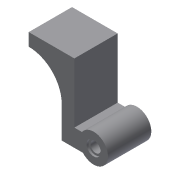
# Autodesk Inventor part: goal holder 2 flipped
Saved by Autodesk Inventor 2015 (Build 190159000, 159)
## iProperties
Created: 2014-11-06
Part Number: goal holder 2 flipped
Material: Generic
Document SubType Name: Modeling
Designer: jesse
Density: 1 g/cm^3
Appearance: Default
Author: jesse
Autodesk Inventor part; units mm, degrees
ref_plane "YZ Plane" through (0, 0, 0) normal (1, 0, 0) x (0, 1, 0)
ref_plane "XZ Plane" through (0, 0, 0) normal (0, 1, 0) x (-1, 0, 0)
ref_plane "XY Plane" through (0, 0, 0) normal (0, 0, 1) x (1, 0, 0)
sketch "Sketch1" plane through (0, 0, 0) normal (0, 0, 1) x (1, 0, 0)
  circle A0 centre (0, 0) radius 11 projected
  circle A1 centre (0, 0) radius 1.75 projected
  circle A2 centre (-8, 0) radius 1.75 projected
  circle A3 centre (0, 8) radius 1.75 projected
  circle A4 centre (8, 0) radius 1.75 projected
  circle A5 centre (0, -8) radius 1.75 projected
extrude "Extrusion1" add sketch "Sketch1" along normal blind 9.525
sketch "Sketch2" plane through (0, 0, 9.525) normal (0, 0, 1) x (1, 0, 0)
  circle A0 centre (0, 0) radius 11 projected
  line L0 (9.0377, 6.2705) -> (14.8574, 6.2705)
  line L1 (14.8574, 6.2705) -> (14.8574, 19.7717)
  line L2 (22.8575, 52.3603) -> (24.5877, 52.3603)
  line L3 (24.5877, 52.3603) -> (24.5877, -7.2164)
  line L4 (24.5877, -7.2164) -> (8.302, -7.2164)
  line L5 (22.8575, 52.3603) -> (14.8574, 52.3603)
  line L6 (14.8574, 19.7717) -> (14.8574, 52.3603)
  point P0 (-11, -11)
  dimension "d11" = 59.5767
  constraints: 14 end point, 3 horizontal, 3 perpendicular, 2 point on circle, 1 parallel, 1 vertical
  measures "d11" distance of L2.end L3.end
extrude "Extrusion2" add sketch "Sketch2" along normal blind 23.8125
mirror "Mirror1" about plane through (0, 0, 0) normal (1, 0, 0) remove original yes
sketch "Sketch3" plane through (-24.5877, -7.2164, 33.3375) normal (0, 0, 1) x (1, 0, 0)
  circle A0 centre (24.5877, 7.2164) radius 3.9688
  dimension "d4" = 7.9375
  constraints: 1 centre point, 1 coincident
  measures "d4" diameter of A0
extrude "Extrusion3" cut sketch "Sketch3" against normal blind 12.4
sketch "Sketch4" plane through (-24.5877, -7.2164, 33.3375) normal (0, 0, 1) x (1, 0, 0)
  circle A0 centre (24.5877, 7.2164) radius 5.5
  dimension "d7" = 11
  constraints: 1 centre point, 1 coincident
  measures "d7" diameter of A0
extrude "Extrusion4" cut sketch "Sketch4" against normal blind 1.5
mirror "Mirror2" about plane through (0, 0, 0) normal (1, 0, 0) remove original yes
sketch "Sketch7" plane through (24.5877, -7.2164, 9.525) normal (1, 0, 0) x (0, 0, -1)
  line L0 (0, 0) -> (0, 59.5767) projected
  line L1 (0, 59.5767) -> (-23.8125, 59.5767) projected
  line L2 (-23.8125, 0) -> (-23.8125, 59.5767) projected
  line L3 (0, 0) -> (-23.8125, 0) projected
  line L4 (0, 59.5767) -> (-23.8125, 59.5767)
  line L5 (-23.8125, 59.5767) -> (-23.8125, 49.8464)
  line L6 (-23.8125, 49.8464) -> (0, 49.8464)
  line L7 (0, 49.8464) -> (0, 59.5767)
  point P0 (9.525, 7.2164)
  dimension "d12" = 9.7303
  constraints: 8 end point, 2 parallel, 1 horizontal, 1 perpendicular, 1 point on line
  measures "d12" distance between parallel lines of L1 L6
extrude "Extrusion5" add sketch "Sketch7" along normal blind 25.4 contours L6 L2 L1 L0
fillet "Fillet3" radius 25.4 1 edges at (24.5877, 42.63, 21.4312)
sketch "Sketch9" plane through (24.5877, -7.2164, 9.525) normal (0, 0, -1) x (-1, 0, 0)
  arc A0 (15.5499, 13.4869) -> (16.2857, 0) centre (24.5877, 7.2164) ccw projected
  line L0 (9.7303, 13.4869) -> (15.5499, 13.4869) projected
  line L1 (9.7303, 59.5767) -> (9.7303, 13.4869) projected
  line L2 (9.7303, 59.5767) -> (-25.4, 59.5767) projected
  line L3 (-25.4, 49.8464) -> (-25.4, 59.5767) projected
  arc A1 (0, 24.4464) -> (-25.4, 49.8464) centre (-25.4, 24.4464) ccw projected
  line L4 (0, 0) -> (0, 24.4464) projected
  line L5 (16.2857, 0) -> (0, 0) projected
extrude "Extrusion6" add sketch "Sketch9" along normal up to surface (9.525 mm away)
mirror "Mirror4" about plane through (0, 0, 0) normal (1, 0, 0) remove original yes
body "Solid1"
